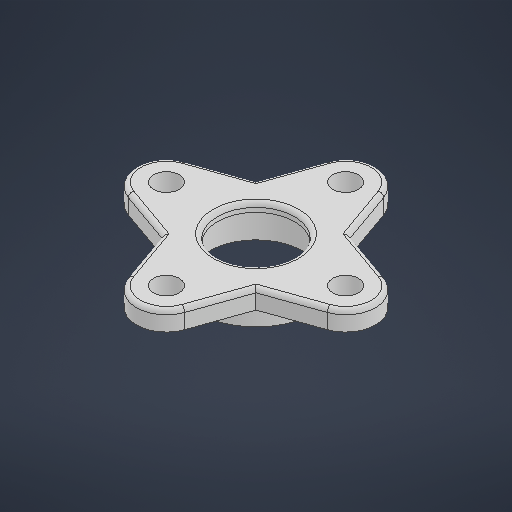
# Autodesk Inventor part: rodamiento_shell
Saved by Autodesk Inventor 2025 (Build 290162010, 162A)
## iProperties
Created: 2024-11-09
Part Number: rodamiento_shell
Material: Generic
Document SubType Name: Modeling
Designer: river
Density: 1 g/cm^3
Appearance: Default
Author: river
Autodesk Inventor part; units mm, degrees
ref_plane "YZ Plane" through (0, 0, 0) normal (1, 0, 0) x (0, 1, 0)
ref_plane "XZ Plane" through (0, 0, 0) normal (0, 1, 0) x (-1, 0, 0)
ref_plane "XY Plane" through (0, 0, 0) normal (0, 0, 1) x (1, 0, 0)
derived "lamina_estator.ipt"
sketch "Sketch3" plane through (0, 3, 0) normal (0, 1, 0) x (1, 0, 0)
  circle A0 centre (-21, 0) radius 3 projected
  line L0 (0, 0) -> (-21, 0) construction
  circle A1 centre (0, -21) radius 3 projected
  circle A2 centre (21, 0) radius 3 projected
  circle A3 centre (0, 0) radius 14 projected
  circle A4 centre (0, 21) radius 3 projected
  circle A5 centre (0, 0) radius 11
  circle A6 centre (-21, 0) radius 7
  circle A7 centre (0, -21) radius 7
  circle A8 centre (21, 0) radius 7
  circle A9 centre (0, 21) radius 7
  line L1 (-4.6667, -13.1993) -> (-23.3333, -6.5997)
  line L2 (-23.3333, 6.5997) -> (-4.6667, 13.1993)
  line L3 (13.1993, -4.6667) -> (6.5997, -23.3333)
  line L4 (-6.5997, -23.3333) -> (-13.1993, -4.6667)
  line L5 (4.6667, 13.1993) -> (23.3333, 6.5997)
  line L6 (23.3333, -6.5997) -> (4.6667, -13.1993)
  line L7 (-13.1993, 4.6667) -> (-6.5997, 23.3333)
  line L8 (6.5997, 23.3333) -> (13.1993, 4.6667)
  circle A10 centre (0, 0) radius 9
  point P0 (-10.9706, -10.9706)
  point P1 (6.5997, -23.3333)
  point P2 (10.9706, -10.9706)
  point P3 (23.3333, 6.5997)
  point P4 (10.9706, 10.9706)
  point P5 (6.5997, 23.3333)
  point P6 (-6.5997, 23.3333)
  point P7 (-10.9706, 10.9706)
  dimension "d1" = 22
  dimension "d2" = 14
  dimension "d5" = 360
  dimension "d9" = 360
  dimension "d15" = 18
  constraints: 16 end point, 6 centre point, 4 point on circle, 4 tangent, 3 coincident, 35 other
  measures "d1" diameter of A5
  measures "d2" diameter of A6
  measures "d15" diameter of A10
extrude "Extrusion1" add sketch "Sketch3" along normal blind 9 contours A3 | A8 L6 L3 A3 | A3 L8 L5 A8 | A8 | A3 L5 L8 | L3 L6 A3 | A3 A9 L8 L5 | L6 L3 A7 A3 | A3 L2 L7 A9 | A9 | A7 L4 L1 A3 | A7 | A3 L7 L2 | L1 L4 A3 | A3 A6 L2 L7 | L4 L1 A6 A3 | A6 | A5
extrude "Extrusion2" cut sketch "Sketch3" along normal blind 4.5 contours A8 L6 L3 A3 | A3 L8 L5 A8 | A8 | A3 L5 L8 | L3 L6 A3 | A3 A9 L8 L5 | L6 L3 A7 A3 | A3 L2 L7 A9 | A9 | A7 L4 L1 A3 | A7 | A3 L7 L2 | L1 L4 A3 | A3 A6 L2 L7 | L4 L1 A6 A3 | A6
extrude "Extrusion3" cut sketch "Sketch3" along normal blind 7 contours A5
fillet "Fillet1" radius 1 13 edges at (-9, 12, 0) (28, 12, 0) (17.1519, 12, 8.7851) (17.1519, 12, -8.7851) (0, 12, -28) (-8.7851, 12, -17.1519) (8.7851, 12, -17.1519) (-28, 12, 0) (-17.1519, 12, 8.7851) (-17.1519, 12, -8.7851) (0, 12, 28) (8.7851, 12, 17.1519) (-8.7851, 12, 17.1519)
body "Solid2"
